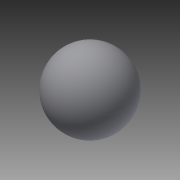
# Autodesk Inventor part: ball
Saved by Autodesk Inventor 2013 (Build 170138000, 138)
## iProperties
Created: 2014-01-21
Part Number: ball
Material: Generic
Document SubType Name: Modeling
Designer: robotics
Density: 1 g/cm^3
Author: robotics
Autodesk Inventor part; units mm, degrees
ref_plane "YZ Plane" through (0, 0, 0) normal (1, 0, 0) x (0, 1, 0)
ref_plane "XZ Plane" through (0, 0, 0) normal (0, 1, 0) x (-1, 0, 0)
ref_plane "XY Plane" through (0, 0, 0) normal (0, 0, 1) x (1, 0, 0)
sketch "Sketch2" plane through (0, 0, 0) normal (0, 1, 0) x (-1, 0, 0)
  circle A0 centre (0, 0) radius 304.8
  line L0 (265.1319, 150.36) -> (-265.1319, -150.36)
  dimension "d1" = 609.6
  constraints: 2 end point, 2 point on circle, 1 centre point, 1 coincident, 1 midpoint
  measures "d1" diameter of A0
revolve "Revolution1" add sketch "Sketch2" angle 360 about axis through (-265.1319, 0, 150.36) along (0.8698552, 0, -0.4933071) picked at (0.1115, 184.6712) contours L0 A0
body "Solid1"
